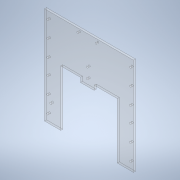
# Autodesk Inventor part: Mech Chassis v7 deckipt
Saved by Autodesk Inventor 2022 (Build 260153000, 153)
## iProperties
Created: 2022-09-25
Part Number: Mech Chassis v7 deckipt
Material: Polycarbonate, Clear
Document SubType Name: Modeling
Designer: matt
Density: 1.2 g/cm^3
Appearance: Polycarbonate - Clear
Mass: 379.99 g
Surface Area: 1114.57 cm^2
Volume: 316.658 cm^3
Author: matt
Autodesk Inventor part; units mm, degrees
ref_plane "YZ Plane" through (0, 0, 0) normal (1, 0, 0) x (0, 1, 0)
ref_plane "XZ Plane" through (0, 0, 0) normal (0, 1, 0) x (-1, 0, 0)
ref_plane "XY Plane" through (0, 0, 0) normal (0, 0, 1) x (1, 0, 0)
sketch "Sketch1" plane through (0, 0, 0) normal (0, 0, 1) x (1, 0, 0)
  circle A0 centre (-10.075, 23.3762) radius 2.8
  circle A1 centre (-10.075, -28.6238) radius 2.8
  circle A2 centre (-10.075, -80.6238) radius 2.8
  circle A3 centre (-10.075, -129.3175) radius 2.8
  circle A4 centre (-10.075, -181.3175) radius 2.8
  circle A5 centre (-10.075, -233.3175) radius 2.8
  circle A6 centre (-269.521, -233.3175) radius 2.8
  circle A7 centre (-269.521, -181.3175) radius 2.8
  circle A8 centre (-269.521, -129.3175) radius 2.8
  circle A9 centre (-269.521, -80.6238) radius 2.8
  circle A10 centre (-269.521, -28.6238) radius 2.8
  circle A11 centre (-269.521, 23.3762) radius 2.8
  line L0 (-279.596, -257.6643) -> (-279.596, 47.723)
  line L1 (0, 47.723) -> (0, -257.6643)
  line L2 (-50.898, -102.277) -> (-50.898, -257.6643)
  line L3 (-228.698, -257.6643) -> (-228.698, -102.277)
  line L4 (0, 47.723) -> (-279.596, 47.723)
  line L5 (-279.596, -257.6643) -> (-228.698, -257.6643)
  line L6 (-50.898, -257.6643) -> (0, -257.6643)
  circle A12 centre (-145.1723, -43.7167) radius 2.8
  circle A13 centre (-175.2462, 34.723) radius 2.75
  circle A14 centre (-118.0962, 34.723) radius 2.75
  circle A15 centre (-260.35, -200.025) radius 3
  line L7 (-123.9223, -92.277) -> (-123.9223, -96.277)
  line L8 (-166.4223, -96.277) -> (-166.4223, -92.277)
  circle A16 centre (-145.1723, -75.7167) radius 2.8
  line L9 (-145.1723, -75.7167) -> (-145.1723, -72.9167) construction
  line L10 (-145.1723, -46.5167) -> (-145.1723, 47.723) construction
  line L11 (-123.9223, -82.277) -> (-123.9223, -92.277)
  line L12 (-166.4223, -82.277) -> (-166.4223, -92.277)
  line L13 (-70.898, -82.277) -> (-123.9223, -82.277)
  line L14 (-166.4223, -82.277) -> (-208.698, -82.277)
  line L15 (-123.9223, -96.277) -> (-166.4223, -96.277)
  line L16 (-73.5425, -10.0701) -> (-115.2306, -10.0701) construction
  line L17 (-73.5425, 1.3522) -> (-115.2306, 1.3522)
  line L18 (-115.2306, -21.4924) -> (-73.5425, -21.4924)
  arc A17 (-73.5425, -21.4924) -> (-73.5425, 1.3522) centre (-73.5425, -10.0701) ccw
  arc A18 (-115.2306, 1.3522) -> (-115.2306, -21.4924) centre (-115.2306, -10.0701) ccw
  line L19 (-216.8021, -10.0701) -> (-175.1139, -10.0701) construction
  line L20 (-216.8021, 1.3522) -> (-175.1139, 1.3522)
  line L21 (-175.1139, -21.4924) -> (-216.8021, -21.4924)
  arc A19 (-216.8021, 1.3522) -> (-216.8021, -21.4924) centre (-216.8021, -10.0701) ccw
  arc A20 (-175.1139, -21.4924) -> (-175.1139, 1.3522) centre (-175.1139, -10.0701) ccw
  arc A21 (-50.898, -102.277) -> (-70.898, -82.277) centre (-70.898, -102.277) ccw
  arc A22 (-208.698, -82.277) -> (-228.698, -102.277) centre (-208.698, -102.277) ccw
  point P0 (-50.898, -82.277)
  point P1 (-228.698, -82.277)
  point P2 (-94.3865, -10.0701)
  point P3 (-195.958, -10.0701)
  dimension "d12" = 5.6
  dimension "d13" = 5.6
  dimension "d2" = 305.3873
  dimension "d3" = 279.596
  dimension "d7" = 5.5
  dimension "d14" = 32
  dimension "d16" = 94.2398
  dimension "d22" = 20
  constraints: 48 end point, 21 centre point, 12 point on circle, 8 tangent, 7 symmetric about line, 6 perpendicular, 5 point on line, 3 horizontal, 2 equal radius, 2 vertical alignment, 1 midpoint, 1 parallel, 7 other
  measures "d2" distance between parallel lines of L6 L4
  measures "d3" distance between parallel lines of L0 L1
  measures "d7" diameter of A13
  measures "d14" distance of L9.start point (-145.172, -43.717)
  measures "d16" distance of L10.start L10.end
  measures "d22" radius of A21
extrude "Extrusion1" add sketch "Sketch1" along normal blind 6.35
body "Solid1"
